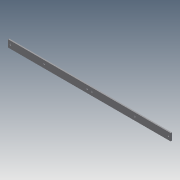
# Autodesk Inventor part: large
Saved by Autodesk Inventor 2011 (Build 150239000, 239)
## iProperties
Created: 2011-12-18
Part Number: large
Document SubType Name: Modeling
Designer: Matthew
Density: 1 g/cm^3
Author: Matthew
Autodesk Inventor part; units mm, degrees
ref_plane "YZ Plane" through (0, 0, 0) normal (1, 0, 0) x (0, 1, 0)
ref_plane "XZ Plane" through (0, 0, 0) normal (0, 1, 0) x (-1, 0, 0)
ref_plane "XY Plane" through (0, 0, 0) normal (0, 0, 1) x (1, 0, 0)
sketch "Sketch1" plane through (0, 0, 0) normal (0, 0, 1) x (1, 0, 0)
  line L0 (-31.9376, 1.7652) -> (399.8624, 1.7652)
  line L1 (399.8624, 1.7652) -> (399.8624, -10.9348)
  line L2 (399.8624, -10.9348) -> (-31.9376, -10.9348)
  line L3 (-31.9376, -10.9348) -> (-31.9376, 1.7652)
  line L4 (183.9624, -4.5848) -> (-26.4766, -4.5848)
  line L5 (-26.4766, -4.5848) -> (394.4014, -4.5848)
  circle A0 centre (-26.4766, -4.5848) radius 1.9812
  circle A1 centre (394.4014, -4.5848) radius 1.9812
  point P0 (0, 0)
  dimension "d0" = 431.8
  dimension "d1" = 12.7
  dimension "d2" = 210.439
  dimension "d3" = 420.878
  dimension "d4" = 3.9624
  dimension "d5" = 3.9624
  constraints: 12 end point, 3 parallel, 2 centre point, 2 coincident, 2 perpendicular, 1 horizontal
  measures "d0" distance of L1.end L2.end
  measures "d1" distance of L0.end L1.end
  measures "d2" distance of L4.start L4.end
  measures "d3" distance of L4.end L5.end
  measures "d4" diameter of A0
  measures "d5" diameter of A1
extrude "Extrusion1" add sketch "Sketch1" along normal blind 3.175
sketch "Sketch2" plane through (-31.9376, 1.7652, 0) normal (0, 1, 0) x (1, 0, 0)
  line L0 (0, -3.175) -> (431.8, -3.175) projected
  line L1 (431.8, 0) -> (431.8, -3.175) projected
  line L2 (0, 0) -> (431.8, 0) projected
  line L3 (0, 0) -> (0, -3.175) projected
  point P0 (31.9376, 0)
extrude "Extrusion2" add sketch "Sketch2" along normal blind 3.175
sketch "Sketch3" plane through (-31.9376, -10.9348, 0) normal (0, -1, 0) x (1, 0, 0)
  line L0 (431.8, 3.175) -> (0, 3.175) projected
  line L1 (0, 0) -> (0, 3.175) projected
  line L2 (431.8, 0) -> (0, 0) projected
  line L3 (431.8, 0) -> (431.8, 3.175) projected
  point P0 (31.9376, 0)
extrude "Extrusion3" add sketch "Sketch3" along normal blind 3.175
sketch "Sketch4" plane through (0, 0, 3.175) normal (0, 0, 1) x (1, 0, 0)
  circle A0 centre (394.4014, -4.5848) radius 1.9812 projected
  circle A1 centre (-26.4766, -4.5848) radius 1.9812 projected
  line L0 (-31.9376, -14.1098) -> (399.8624, -14.1098) projected
  line L1 (394.4014, -4.5848) -> (298.7704, -4.5848)
  line L2 (-26.4766, -4.5848) -> (69.1544, -4.5848)
  circle A2 centre (69.1544, -4.5848) radius 1.9812
  circle A3 centre (298.7704, -4.5848) radius 1.9812
  point P0 (0, 0)
  dimension "d12" = 95.631
  dimension "d13" = 95.631
  constraints: 4 end point, 2 centre point, 2 coincident, 1 collinear, 1 parallel
  measures "d12" distance of L1.start L1.end
  measures "d13" distance of L2.start L2.end
extrude "Extrusion4" cut sketch "Sketch4" against normal blind 25.4 contours A3 | A2
sketch "Sketch5" plane through (0, 0, 0) normal (0, 0, -1) x (-1, 0, 0)
  circle A0 centre (-298.7704, -4.5848) radius 1.9812 projected
  point P0 (0, 0)
extrude "Extrusion5" add sketch "Sketch5" against normal blind 3.175
sketch "Sketch6" plane through (0, 0, 0) normal (0, 0, -1) x (-1, 0, 0)
  circle A0 centre (-69.1544, -4.5848) radius 1.9812 projected
  point P0 (0, 0)
extrude "Extrusion6" add sketch "Sketch6" against normal blind 3.175
sketch "Sketch7" plane through (0, 0, 0) normal (0, 0, -1) x (-1, 0, 0)
  circle A0 centre (-394.4014, -4.5848) radius 1.9812 projected
  circle A1 centre (26.4766, -4.5848) radius 1.9812 projected
  line L0 (31.9376, 4.9402) -> (-399.8624, 4.9402) projected
  line L1 (26.4766, -4.5848) -> (-63.1854, -4.5848)
  line L2 (-394.4014, -4.5848) -> (-304.7394, -4.5848)
  circle A2 centre (-304.7394, -4.5848) radius 1.9812
  circle A3 centre (-63.1854, -4.5848) radius 1.9812
  point P0 (0, 0)
  dimension "d20" = 89.662
  dimension "d21" = 89.662
  constraints: 4 end point, 2 centre point, 2 coincident, 1 collinear, 1 parallel
  measures "d20" distance of L1.start L1.end
  measures "d21" distance of L2.start L2.end
extrude "Extrusion7" cut sketch "Sketch7" against normal blind 3.175 contours A2 | A3
sketch "Sketch8" plane through (0, 0, 3.175) normal (0, 0, 1) x (1, 0, 0)
  circle A0 centre (63.1854, -4.5848) radius 1.9812 projected
  circle A1 centre (304.7394, -4.5848) radius 1.9812 projected
  circle A2 centre (394.4014, -4.5848) radius 1.9812 projected
  circle A3 centre (-26.4766, -4.5848) radius 1.9812 projected
  point P0 (0, 0)
extrude "Extrusion8" add sketch "Sketch8" against normal blind 3.175
sketch "Sketch9" plane through (0, 0, 3.175) normal (0, 0, 1) x (1, 0, 0)
  line L0 (-31.9376, -14.1098) -> (399.8624, -14.1098) projected
  line L1 (183.9624, -4.5848) -> (304.2314, -4.5848)
  line L2 (304.2314, -4.5848) -> (63.6934, -4.5848)
  circle A0 centre (304.2314, -4.5848) radius 1.9812
  circle A1 centre (63.6934, -4.5848) radius 1.9812
  line L3 (304.2314, -4.5848) -> (393.8934, -4.5848)
  line L4 (63.6934, -4.5848) -> (-25.9686, -4.5848)
  circle A2 centre (393.8934, -4.5848) radius 1.9812
  circle A3 centre (-25.9686, -4.5848) radius 1.9812
  point P0 (0, 0)
  dimension "d26" = 120.269
  dimension "d27" = 240.538
  dimension "d28" = 3.9624
  dimension "d29" = 89.662
  dimension "d30" = 89.662
  constraints: 8 end point, 4 centre point, 4 coincident, 2 collinear, 1 parallel, 1 point on line
  measures "d26" distance of L1.start L1.end
  measures "d27" distance of L1.end L2.end
  measures "d28" diameter of A0
  measures "d29" distance of L3.start L3.end
  measures "d30" distance of L4.start L4.end
extrude "Extrusion9" cut sketch "Sketch9" against normal blind 3.175
sketch "Sketch10" plane through (0, 0, 0) normal (0, 0, -1) x (-1, 0, 0)
  line L0 (31.9376, 4.9402) -> (-399.8624, 4.9402) projected
  line L1 (-183.9624, -4.5848) -> (-177.6124, -4.5848)
  line L2 (-177.6124, -4.5848) -> (-190.3124, -4.5848)
  circle A0 centre (-177.6124, -4.5848) radius 1.9812
  circle A1 centre (-190.3124, -4.5848) radius 1.9812
  point P0 (0, 0)
  dimension "d33" = 6.35
  dimension "d34" = 12.7
  constraints: 4 end point, 2 centre point, 2 coincident, 1 collinear, 1 parallel
  measures "d33" distance of L1.start L1.end
  measures "d34" distance of L1.end L2.end
extrude "Extrusion10" cut sketch "Sketch10" against normal blind 3.175
body "Solid1"
